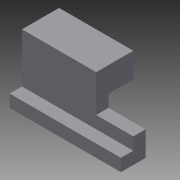
# Autodesk Inventor part: 4.1e Q4
Saved by Autodesk Inventor 2015 (Build 190159000, 159)
## iProperties
Created: 2017-11-15
Part Number: 4.1e Q4
Material: Generic
Document SubType Name: Modeling
Designer: Administrator
Density: 1 g/cm^3
Appearance: Default
Author: Administrator
Autodesk Inventor part; units mm, degrees
ref_plane "YZ Plane" through (0, 0, 0) normal (1, 0, 0) x (0, 1, 0)
ref_plane "XZ Plane" through (0, 0, 0) normal (0, 1, 0) x (-1, 0, 0)
ref_plane "XY Plane" through (0, 0, 0) normal (0, 0, 1) x (1, 0, 0)
sketch "Sketch1" plane through (0, 0, 0) normal (0, 0, 1) x (1, 0, 0)
  line L0 (0, 0) -> (0, 63.5)
  line L1 (0, 63.5) -> (76.2, 63.5)
  line L2 (76.2, 63.5) -> (76.2, 25.4)
  line L3 (76.2, 25.4) -> (114.3, 25.4)
  line L4 (114.3, 25.4) -> (114.3, 0)
  line L5 (114.3, 0) -> (0, 0)
  dimension "d0" = 63.5
  dimension "d1" = 114.3
  dimension "d2" = 25.4
  dimension "d3" = 76.2
  constraints: 12 end point, 5 perpendicular, 1 vertical
  measures "d0" distance of L0.start L0.end
  measures "d1" distance of L4.end L0.start
  measures "d2" distance of L3.end L4.end
  measures "d3" distance of L0.end L1.end
extrude "Extrusion1" add sketch "Sketch1" along normal blind 38.1
sketch "Sketch2" plane through (0, 0, 38.1) normal (0, 0, 1) x (1, 0, 0)
  line L0 (0, 63.5) -> (0, 0) projected
  line L1 (0, 12.7) -> (114.3, 12.7)
  line L2 (114.3, 12.7) -> (114.3, 0)
  line L3 (114.3, 0) -> (0, 0)
  line L4 (0, 0) -> (114.3, 0) projected
  line L5 (0, 0) -> (0, 12.7)
  dimension "d6" = 114.3
  dimension "d7" = 12.7
  constraints: 8 end point, 2 collinear, 1 horizontal, 1 point on line
  measures "d6" distance of L1.start L1.end
  measures "d7" distance of L1.end L2.end
extrude "Extrusion2" add sketch "Sketch2" along normal blind 12.7
sketch "Sketch3" plane through (114.3, 0, 0) normal (1, 0, 0) x (0, 0, -1)
  line L0 (-25.4, 38.1) -> (-25.4, 0)
  line L1 (-25.4, 0) -> (0, 0)
  line L2 (0, 0) -> (-50.8, 0) projected
  line L3 (0, 0) -> (0, 38.1)
  line L4 (0, 63.5) -> (0, 25.4) projected
  line L5 (-25.4, 38.1) -> (0, 38.1)
  line L6 (0, 0) -> (-25.4, 0)
  dimension "d10" = 25.4
  dimension "d11" = 38.1
  constraints: 10 end point, 2 collinear, 1 perpendicular, 1 point on line, 1 vertical
  measures "d10" distance of L0.start L3.end
  measures "d11" distance of L1.end L3.end
extrude "Extrusion3" cut sketch "Sketch3" against normal blind 150.8125
body "Solid1"
